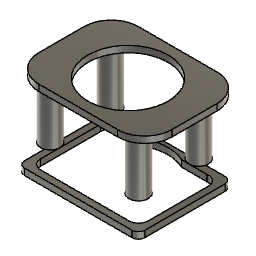
suporte joystick (Autodesk Fusion 360 design; units mm, degrees)
Autodesk Fusion 360 part; units mm, degrees
sketch "Esboço1" plane through (0, 0, 0) normal (0, 0, 1) x (1, 0, 0)
  circle A0 centre (0, 0) radius 12.5
  line L0 (0, 0) -> (0, 8.3) construction
  line L1 (0, 8.3) -> (13.8, 8.3) construction
  line L2 (0, 0) -> (0, -10.5) construction
  line L3 (0, -10.5) -> (13.8, -10.5) construction
  circle A1 centre (13.8, 8.3) radius 1.5
  circle A2 centre (13.8, -10.5) radius 1.5
  circle A3 centre (-13.8, 8.3) radius 1.5
  circle A4 centre (-13.8, -10.5) radius 1.5
  circle A5 centre (13.8, 8.3) radius 3
  circle A6 centre (13.8, -10.5) radius 3
  circle A7 centre (-13.8, 8.3) radius 3
  circle A8 centre (-13.8, -10.5) radius 3
  line L4 (18.5, 13.25) -> (-18.5, 13.25) construction
  line L5 (-18.5, 13.25) -> (-18.5, -13.25) construction
  line L6 (-18.5, -13.25) -> (18.5, -13.25) construction
  line L7 (18.5, -13.25) -> (18.5, 13.25) construction
  line L8 (18.5, 13.25) -> (-18.5, -13.25) construction
  line L9 (-18.5, 13.25) -> (18.5, -13.25) construction
  line L10 (-18.8, -13.55) -> (18.8, -13.55)
  line L11 (18.8, -13.55) -> (18.8, 13.55)
  line L12 (18.8, 13.55) -> (-18.8, 13.55)
  line L13 (-18.8, 13.55) -> (-18.8, -13.55)
  line L14 (-20.8, 15.55) -> (-20.8, -15.55)
  line L15 (-20.8, -15.55) -> (20.8, -15.55)
  line L16 (20.8, -15.55) -> (20.8, 15.55)
  line L17 (20.8, 15.55) -> (-20.8, 15.55)
  dimension "d1" = 25
  dimension "d2" = 8.3
  dimension "d3" = 13.8
  dimension "d4" = 10.5
  dimension "d5" = 13.8
  dimension "d6" = 3
  dimension "d7" = 3
  dimension "d8" = 6
  dimension "d9" = 6
  dimension "d10" = 26.5
  dimension "d11" = 37
  dimension "d12" = 0.3
  dimension "d13" = 2.3
  constraint coincident A0.centre L0.start
  constraint vertical L0
  constraint perpendicular L0 L1
  constraint parallel L0 L2
  constraint perpendicular L2 L3
  constraint coincident L1.end A1.centre
  constraint coincident L3.end A2.centre
  constraint symmetric L2 A1 A3
  constraint symmetric L2 A2 A4
  constraint concentric A1 A5
  constraint concentric A2 A6
  constraint symmetric L0 A5 A7
  constraint symmetric L0 A6 A8
  constraint horizontal L4
  constraint perpendicular L4 L5
  constraint parallel L4 L6
  constraint parallel L5 L7
  constraint coincident L8 A0.centre
  constraint coincident L9 A0.centre
  measures "d1" diameter of A0
  measures "d2" distance of A0.centre L0.end
  measures "d3" distance of L0.end L1.end
  measures "d4" distance of A0.centre L2.end
  measures "d5" distance of L2.end L3.end
  measures "d6" diameter of A1
  measures "d7" diameter of A2
  measures "d8" diameter of A5
  measures "d9" diameter of A6
  measures "d10" distance of L4.end L5.end
  measures "d11" distance of L5.end L6.end
extrude "Extrusão1" add sketch "Esboço1" along normal blind 2 contours A5 | A6 | A7 | A8 | L10 L11 L12 L13 | L14 L15 L16 L17 makes body 1
sketch "Esboço2" plane through (0, 0, 0) normal (0, 0, -1) x (1, 0, 0)
  circle A0 centre (13.8, 10.5) radius 1.5
  circle A1 centre (-13.8, -8.3) radius 1.5
  circle A2 centre (13.8, -8.3) radius 1.5
  circle A3 centre (0, 0) radius 12.5
  circle A4 centre (-13.8, 10.5) radius 1.5
  line L0 (-20.8, -15.55) -> (20.8, -15.55)
  line L1 (20.8, -15.55) -> (20.8, 15.55)
  line L2 (20.8, 15.55) -> (-20.8, 15.55)
  line L3 (-20.8, 15.55) -> (-20.8, -15.55)
  circle A5 centre (-13.8, -8.3) radius 3
  circle A6 centre (-13.8, 10.5) radius 3
  circle A7 centre (13.8, 10.5) radius 3
  circle A8 centre (13.8, -8.3) radius 3
  line L4 (-12.6319, 9.559) -> (12.6319, 9.559) construction
  line L5 (12.6319, 9.559) -> (12.6319, -9.559) construction
  line L6 (12.6319, -9.559) -> (-12.6319, -9.559) construction
  line L7 (-12.6319, -9.559) -> (-12.6319, 9.559) construction
  line L8 (-12.6319, 9.559) -> (12.6319, -9.559) construction
  line L9 (12.6319, 9.559) -> (-12.6319, -9.559) construction
  line L10 (-14.9047, 11.5147) -> (14.9047, 11.5147) construction
  line L11 (14.9047, 11.5147) -> (14.9047, -11.5147) construction
  line L12 (14.9047, -11.5147) -> (-14.9047, -11.5147) construction
  line L13 (-14.9047, -11.5147) -> (-14.9047, 11.5147) construction
  line L14 (-14.9047, 11.5147) -> (14.9047, -11.5147) construction
  line L15 (14.9047, 11.5147) -> (-14.9047, -11.5147) construction
  dimension "d16" = 6
  dimension "d17" = 6
  dimension "d18" = 6
  dimension "d19" = 6
  constraint concentric A1 A5
  constraint concentric A4 A6
  constraint concentric A0 A7
  constraint concentric A2 A8
  constraint horizontal L4
  constraint perpendicular L4 L5
  constraint parallel L4 L6
  constraint parallel L5 L7
  constraint coincident L8 A3.centre
  constraint coincident L9 A3.centre
  constraint coincident A4 L4.start
  constraint coincident A3.centre origin
  constraint horizontal L10
  constraint perpendicular L10 L11
  constraint parallel L10 L12
  constraint parallel L11 L13
  constraint coincident L14 A3.centre
  constraint coincident L15 A3.centre
  constraint coincident A4 L10.start
  measures "d16" diameter of A5
  measures "d17" diameter of A6
  measures "d18" diameter of A7
  measures "d19" diameter of A8
extrude "Extrusão2" add sketch "Esboço2" along normal blind 17 contours A5 | A6 | A7 | A8 bodies 1
extrude "Extrusão3" add 1 faces at (19.4222, 2.4719, 0) along direction (0, 0, -1) blind 2 from surface at 10 separate body on bodies 1 makes body 2
sketch "Esboço3" plane through (0, 0, -12) normal (0, 0, -1) x (1, 0, 0)
  circle A0 centre (13.8, -8.3) radius 3
  circle A1 centre (13.8, 10.5) radius 3
  circle A2 centre (-13.8, -8.3) radius 3
  circle A3 centre (-13.8, 10.5) radius 3
  circle A4 centre (0, 0) radius 12.5
  line L0 (-20.8, -15.55) -> (20.8, -15.55)
  line L1 (20.8, -15.55) -> (20.8, 15.55)
  line L2 (20.8, 15.55) -> (-20.8, 15.55)
  line L3 (-20.8, 15.55) -> (-20.8, -15.55)
  line L4 (16.8, -8.3) -> (16.8, 10.5)
  line L5 (14.1944, -11.274) -> (-14.1944, -11.274)
  line L6 (0, 0) -> (0, -3)
  line L7 (0, 0) -> (-4, 0)
  line L8 (13.9881, 13.4941) -> (-13.7994, 13.5)
  line L9 (-16.7992, -8.371) -> (-16.8, 10.4999)
  line L10 (18.8, 13.55) -> (-18.8, 13.55)
  line L11 (-18.8, 13.55) -> (-18.8, -13.55)
  line L12 (-18.8, -13.55) -> (18.8, -13.55)
  line L13 (18.8, -13.55) -> (18.8, 13.55)
  line L14 (18.8, 13.55) -> (18.8, 15.55)
  line L15 (18.8, 15.55) -> (-19, 15.55)
  line L16 (-18.8, 13.55) -> (-18.8, 15.7823)
  dimension "d25" = -2
  constraint coincident A0 L4.start
  constraint tangent A0 L4
  constraint coincident A1 L4.end
  constraint tangent A1 L4
  constraint coincident A0 L5.start
  constraint coincident A2 L5.end
  constraint horizontal L5
  constraint coincident A4.centre L6.start
  constraint parallel L1 L6
  constraint parallel L5 L7
  constraint coincident A1 L8.start
  constraint coincident A3 L8.end
  constraint tangent A3 L8
  constraint coincident A2 L9.start
  constraint coincident A3 L9.end
  constraint tangent A3 L9
  constraint coincident L2 L14.end
  constraint perpendicular L2 L14
  constraint coincident L2 L15.end
  constraint perpendicular L11 L15
  constraint perpendicular L15 L16
extrude "Extrusão4" cut sketch "Esboço3" against normal blind 2 contours A0 A1 A2 A3 A4 L4 L5 L8 L9 | L0 L1 L2 L3 L11 L12 L13 L14 L15 L16 bodies 2
move_body "Mover1" bodies 2 to x (1, 0, 0) y (0, 1, 0) z (0, 0, 1) at (0, 0, -13)
fillet "Arredondamento1" radius 8.5 4 edges at (20.8, -15.55, 1) (-20.8, -15.55, 1) (20.8, 15.55, 1) (-20.8, 15.55, 1) on bodies 1
fillet "Arredondamento2" radius 2 4 edges at (-18.8, 13.55, -24) (18.8, 13.55, -24) (-18.8, -15.55, -24) (18.8, -15.55, -24) on bodies 2
sketch "Esboço4" plane through (0, 0, 2) normal (0, 0, 1) x (-1, 0, 0)
  arc A0 (12.3, -15.55) -> (20.8, -7.05) centre (12.3, -7.05) ccw
  line L0 (20.8, -7.05) -> (20.8, 7.05)
  arc A1 (20.8, 7.05) -> (12.3, 15.55) centre (12.3, 7.05) ccw
  line L1 (12.3, 15.55) -> (-12.3, 15.55)
  arc A2 (-12.3, 15.55) -> (-20.8, 7.05) centre (-12.3, 7.05) ccw
  line L2 (-20.8, 7.05) -> (-20.8, -7.05)
  arc A3 (-20.8, -7.05) -> (-12.3, -15.55) centre (-12.3, -7.05) ccw
  line L3 (-12.3, -15.55) -> (12.3, -15.55)
  circle A4 centre (-13.8, 10.5) radius 1.5
  circle A5 centre (13.8, -8.3) radius 1.5
  circle A6 centre (-13.8, -8.3) radius 1.5
  circle A7 centre (0, 0) radius 12.5
  circle A8 centre (13.8, 10.5) radius 1.5
extrude "Extrusão5" add sketch "Esboço4" against normal blind 8 contours A4 | A5 | A6 | A8 bodies 1
